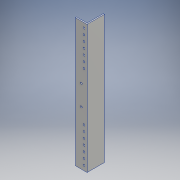
# Autodesk Inventor part: bepf_podwozie_belka_glowna
Saved by Autodesk Inventor 2017 (Build 210142000, 142)
## iProperties
Created: 2016-11-24
Part Number: bepf_podwozie_belka_glowna
Material: Aluminium 6061
Document SubType Name: Modeling
Designer: gagato
Density: 2.7 g/cm^3
Appearance: Aluminium — płaski
Mass: 56.3291 g
Surface Area: 222.563 cm^2
Volume: 20.8626 cm^3
Author: gagato
Autodesk Inventor part; units mm, degrees
ref_plane "YZ Plane" through (0, 0, 0) normal (1, 0, 0) x (0, 1, 0)
ref_plane "XZ Plane" through (0, 0, 0) normal (0, 1, 0) x (-1, 0, 0)
ref_plane "XY Plane" through (0, 0, 0) normal (0, 0, 1) x (1, 0, 0)
sketch "Szkic1" plane through (0, 0, 0) normal (0, 0, 1) x (1, 0, 0)
  line L0 (0, 0) -> (0, 30)
  line L1 (0, 30) -> (-2, 30)
  line L2 (-2, 30) -> (-2, 2)
  line L3 (-2, 2) -> (-20, 2)
  line L4 (-20, 2) -> (-20, 0)
  line L5 (-20, 0) -> (0, 0)
  dimension "d0" = 30
  dimension "d1" = 2
  dimension "d2" = 28
  dimension "d4" = 20
  constraints: 12 end point, 4 perpendicular, 2 vertical
  measures "d0" distance of L0.start L0.end
  measures "d1" distance of L0.end L1.end
  measures "d2" distance of L1.end L2.end
  measures "d4" distance of L4.end L0.start
extrude "Wyciągnięcie proste1" add sketch "Szkic1" along normal mid plane 220
sketch "Szkic2" plane through (-20, 2, 110) normal (0, 1, 0) x (1, 0, 0)
  line L0 (18, 0) -> (0, 0) projected
  line L1 (20, 0) -> (20, 220) projected
  point P0 (20, 110)
  point P1 (14.8, 8.1)
  dimension "d7" = 8.1
  dimension "d8" = 5.2
  measures "d7" distance from line of L0 point (14.8, 8.1)
  measures "d8" distance from line of point (14.8, 8.1) L1
hole "Otwór1" at (-5.2, 2, 101.9) direction (0, -1, 0) diameter 3.2 end through all
pattern_linear "Szyk prostokątny1" count 7 spacing 10 along (0, 0, -1) of "Otwór1"
mirror "Odbij1" about plane through (0, 0, 0) normal (0, 0, 1) of "Otwór1", "Szyk prostokątny1"
sketch "Szkic3" plane through (-20, 2, 110) normal (0, 1, 0) x (1, 0, 0)
  line L0 (24, 110) -> (-4, 110) projected
  line L1 (10, 127.5) -> (10, 92.5) construction
  line L2 (20, 220) -> (20, 0) projected
  point P0 (20, 110)
  point P1 (10, 110)
  dimension "d19" = 35
  dimension "d20" = 10
  constraints: 2 coincident, 2 end point, 2 midpoint, 1 vertical
  measures "d19" distance of L1.start L1.end
  measures "d20" distance between parallel lines of L2 L1
hole "Otwór2" at (-10, 2, -17.5) at (-10, 2, 17.5) direction (0, -1, 0) diameter 3.2 end through all
